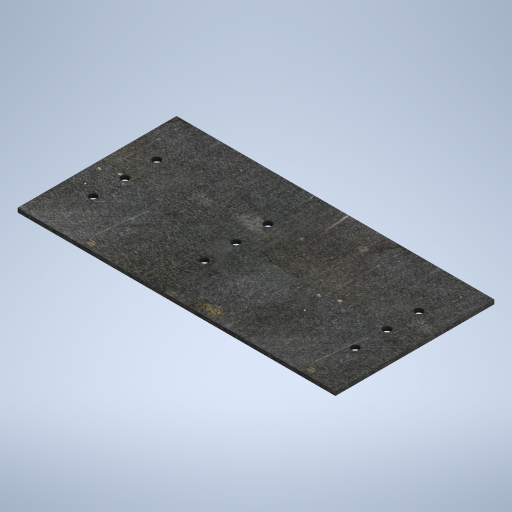
# Autodesk Inventor part: Wedge_piece1
Saved by Autodesk Inventor 2023 (Build 270158000, 158)
## iProperties
Created: 2022-12-26
Part Number: Wedge_piece1
Material: Steel
Document SubType Name: Modeling
Designer: justi
Density: 7.85 g/cm^3
Appearance: Plate
Mass: 102.419 g
Surface Area: 669.353 cm^2
Volume: 102.419 cm^3
Author: justi
Autodesk Inventor part; units mm, degrees
ref_plane "YZ Plane" through (0, 0, 0) normal (1, 0, 0) x (0, 1, 0)
ref_plane "XZ Plane" through (0, 0, 0) normal (0, 1, 0) x (-1, 0, 0)
ref_plane "XY Plane" through (0, 0, 0) normal (0, 0, 1) x (1, 0, 0)
sketch "Sketch1" plane through (0, 0, 0) normal (0, 1, 0) x (-1, 0, 0)
  line L0 (0, 0) -> (-254, 0)
  line L1 (-254, 0) -> (-254, -127)
  line L2 (-254, -127) -> (0, -127)
  line L3 (0, -127) -> (0, 0)
  dimension "d0" = 254
  dimension "d3" = 127
  constraints: 8 end point, 2 parallel, 1 horizontal, 1 perpendicular
  measures "d0" distance of L1.end L2.end
  measures "d3" distance of L0.end L1.end
extrude "Extrusion1" add sketch "Sketch1" along normal blind 3.175
sketch "Sketch2" plane through (0, 3.175, 0) normal (0, 1, 0) x (1, 0, 0)
  circle A0 centre (22.225, 88.9) radius 3.175
  circle A1 centre (22.225, 63.5) radius 3.175
  circle A2 centre (22.225, 38.1) radius 3.175
  line L0 (0, 127) -> (0, 0) projected
  circle A3 centre (231.775, 63.5) radius 3.175
  circle A4 centre (231.775, 88.9) radius 3.175
  circle A5 centre (231.775, 38.1) radius 3.175
  line L1 (254, 0) -> (254, 127) projected
  circle A6 centre (111.125, 88.9) radius 3.175
  circle A7 centre (111.125, 63.5) radius 3.175
  circle A8 centre (111.125, 38.1) radius 3.175
  point P0 (0, 63.5)
  point P1 (254, 63.5)
  point P2 (0, 63.5)
  dimension "d4" = 6.35
  dimension "d5" = 6.35
  dimension "d6" = 6.35
  dimension "d7" = 22.225
  dimension "d8" = 22.225
  dimension "d9" = 22.225
  dimension "d10" = 25.4
  dimension "d11" = 25.4
  dimension "d12" = 0
  dimension "d13" = 6.35
  dimension "d14" = 6.35
  dimension "d15" = 6.35
  dimension "d16" = 22.225
  dimension "d17" = 22.225
  dimension "d18" = 22.225
  dimension "d19" = 0
  dimension "d20" = 25.4
  dimension "d21" = 25.4
  dimension "d22" = 6.35
  dimension "d23" = 6.35
  dimension "d24" = 6.35
  dimension "d25" = 111.125
  dimension "d26" = 111.125
  dimension "d27" = 111.125
  dimension "d28" = 0
  dimension "d29" = 25.4
  dimension "d30" = 25.4
  constraints: 9 centre point, 3 midpoint
  measures "d4" diameter of A0
  measures "d5" diameter of A1
  measures "d6" diameter of A2
  measures "d7" distance from line of L0 A0.centre
  measures "d8" distance from line of L0 A1.centre
  measures "d9" distance from line of L0 A2.centre
  measures "d10" distance of A1.centre A0.centre
  measures "d11" distance of A2.centre A1.centre
  measures "d12" vertical distance of point (0, 63.5) A1.centre
  measures "d13" diameter of A3
  measures "d14" diameter of A4
  measures "d15" diameter of A5
  measures "d16" distance from line of L1 A4.centre
  measures "d17" distance from line of L1 A3.centre
  measures "d18" distance from line of L1 A5.centre
  measures "d19" vertical distance of point (254, 63.5) A3.centre
  measures "d20" distance of A3.centre A4.centre
  measures "d21" distance of A3.centre A5.centre
  measures "d22" diameter of A6
  measures "d23" diameter of A7
  measures "d24" diameter of A8
  measures "d25" distance from line of L0 A6.centre
  measures "d26" distance from line of L0 A7.centre
  measures "d27" distance from line of L0 A8.centre
  measures "d28" vertical distance of point (0, 63.5) A7.centre
  measures "d29" distance of A6.centre A7.centre
  measures "d30" distance of A7.centre A8.centre
extrude "Extrusion2" cut sketch "Sketch2" against normal blind 3.175
body "Solid1"
